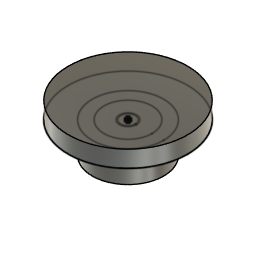
Neck piece v1 (Autodesk Fusion 360 design; units mm, degrees)
Autodesk Fusion 360 part; units mm, degrees
sketch "Sketch1" plane through (0, 0, 0) normal (0, 0, 1) x (1, 0, 0)
  circle A0 centre (0, 0) radius 14.95
  circle A1 centre (0, 0) radius 10.05
  circle A2 centre (0, 0) radius 3.05
  circle A3 centre (0, 0) radius 3.55
  circle A4 centre (0, 0) radius 25
  dimension "d1" = 29.9
  dimension "d2" = 20.1
  dimension "d7" = 6.1
  dimension "d8" = 7.1
  dimension "d9" = 50
  constraint coincident A0.centre A1.centre
  constraint concentric A0 A1
  constraint concentric A0 A2
  constraint concentric A0 A3
  measures "d1" diameter of A0
  measures "d2" diameter of A1
  measures "d7" diameter of A2
  measures "d8" diameter of A3
  measures "d9" diameter of A4
extrude "Extrude1" add sketch "Sketch1" against normal blind 13 contours A0
extrude "Extrude2" add sketch "Sketch1" against normal blind 7 contours A1 | A2 | A3
extrude "Extrude3" add sketch "Sketch1" against normal blind 8 contours A3
extrude "Extrude4" cut 1 faces at (3.3701, -0.1764, -8) along direction (0, 0, 1) blind 1.5
extrude "Extrude5" add sketch "Sketch1" along normal blind 7 contours A0 | A1 | A2 | A3 | A4
